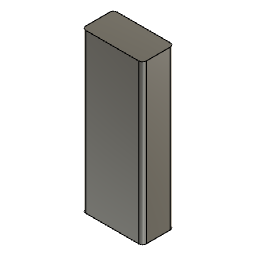
AirQuam v21 (Autodesk Fusion 360 archive; units mm, degrees)
design "powerbank"
Autodesk Fusion 360 part; units mm, degrees
sketch "Sketch1" plane through (0, 0, 0) normal (0, 0, 1) x (1, 0, 0)
  line L0 (-18, -11) -> (18, -11)
  arc A0 (18, -11) -> (18, 11) centre (18, 0) ccw
  line L1 (18, 11) -> (-18, 11)
  arc A1 (-18, 11) -> (-18, -11) centre (-18, 0) ccw
  line L2 (-29, 0) -> (29, 0) construction
  line L3 (19.5, -10.15) -> (-19.5, -10.15)
  line L4 (-19.5, -10.15) -> (-19.5, 10.15)
  line L5 (-19.5, 10.15) -> (19.5, 10.15)
  line L6 (19.5, 10.15) -> (19.5, -10.15)
  line L7 (19.5, -10.15) -> (-19.5, 10.15) construction
  line L8 (-19.5, -10.15) -> (19.5, 10.15) construction
  dimension "d5" = 58
  dimension "d6" = 22
  dimension "d7" = 20.3
  dimension "d8" = 39
  constraint tangent L0 A0
  constraint tangent A0 L1
  constraint parallel L0 L1
  constraint tangent L1 A1
  constraint tangent L0 A1
  constraint midpoint A1 L2.start
  constraint midpoint A0 L2.end
  constraint horizontal L2
  constraint perpendicular L3 L4
  constraint parallel L3 L5
  constraint parallel L4 L6
  constraint horizontal L3
  constraint coincident L7 origin
  constraint coincident L8 origin
  constraint midpoint L2 origin
  measures "d5" distance of L2.start L2.end
  measures "d6" distance of L0 L1
  measures "d7" distance of L3.end L4.end
  measures "d8" distance of L4.end L5.end
extrude "Extrude1" add sketch "Sketch1" along normal blind 50 and the other way blind 52 contours L3 L4 L5 L6
fillet "Fillet1" radius 2.5 4 edges at (19.5, -10.15, -1) (-19.5, -10.15, -1) (19.5, 10.15, -1) (-19.5, 10.15, -1)
